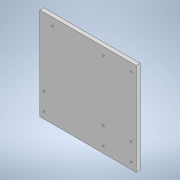
# Autodesk Inventor part: newMATXMount
Saved by Autodesk Inventor 2020 (Build 240168000, 168)
## iProperties
Created: 2026-07-11
Part Number: newMATXMount
Material: Generic
Document SubType Name: Modeling
Designer: Nessa
Density: 1 g/cm^3
Appearance: Default
Author: Nessa
Autodesk Inventor part; units mm, degrees
ref_plane "YZ Plane" through (0, 0, 0) normal (1, 0, 0) x (0, 1, 0)
ref_plane "XZ Plane" through (0, 0, 0) normal (0, 1, 0) x (-1, 0, 0)
ref_plane "XY Plane" through (0, 0, 0) normal (0, 0, 1) x (1, 0, 0)
sketch "Sketch1" plane through (0, 0, 0) normal (0, 0, 1) x (1, 0, 0)
  line L0 (-125, 120) -> (125, 120)
  line L1 (125, 120) -> (125, -120)
  line L2 (125, -120) -> (-125, -120)
  line L3 (-125, -120) -> (-125, 120)
  point P0 (0, 0)
  dimension "d0" = 250
  dimension "d1" = 240
  dimension "d2" = 125
  dimension "d3" = 120
  constraints: 8 end point, 2 parallel, 1 horizontal, 1 perpendicular
  measures "d0" distance of L1.end L2.end
  measures "d1" distance of L0.end L1.end
  measures "d2" distance from line of L3 point (0, 0)
  measures "d3" distance from line of L0 point (0, 0)
extrude "Extrusion1" add sketch "Sketch1" along normal mid plane 10
sketch "Sketch5" plane through (0, 0, 5) normal (0, 0, 1) x (1, 0, 0)
  line L0 (-115, 100) -> (-115, -103.2)
  line L1 (-92.14, 100) -> (-92.14, -103.2)
  line L2 (39.94, 100) -> (39.94, -103.2)
  line L3 (112.33, 100) -> (112.33, -103.2)
  line L4 (-92.14, 100) -> (112.33, 100)
  line L5 (-115, -57.48) -> (39.94, -57.48)
  line L6 (112.33, -57.48) -> (39.94, -57.48)
  line L7 (-115, -103.2) -> (39.94, -103.2)
  line L8 (112.33, -103.2) -> (39.94, -103.2)
  line L9 (-115, 100) -> (-92.14, 100)
  line L10 (-125, 120) -> (-125, -120) projected
  line L11 (125, 120) -> (-125, 120) projected
  point P0 (0, 0)
  dimension "d25" = 10
  dimension "d26" = 22.86
  dimension "d27" = 72.39
  dimension "d28" = 132.08
  dimension "d29" = 45.72
  dimension "d30" = 157.48
  dimension "d38" = 20
  constraints: 20 end point, 6 point on line, 4 perpendicular, 4 vertical, 2 collinear, 1 horizontal, 1 parallel
  measures "d25" distance between parallel lines of L10 L0
  measures "d26" distance between parallel lines of L1 L0
  measures "d27" distance between parallel lines of L3 L2
  measures "d28" distance between parallel lines of L2 L1
  measures "d29" distance between parallel lines of L8 L6
  measures "d30" distance between parallel lines of L4 L6
  measures "d38" distance between parallel lines of L11 L4
hole "Hole2" at (-92.14, 100, 5) at (39.94, 100, 5) at (112.33, 100, 5) at (112.33, -57.48, 5) at (39.94, -57.48, 5) at (39.94, -103.2, 5) at (112.33, -103.2, 5) at (-115, -57.48, 5) at (-115, -103.2, 5) direction (0, 0, -1) diameter 3.6 depth 5 tip angle 118
equation "\"d2\" = 0.5 * d0"
equation "\"d3\" = 0.5 * d1"
body "Solid1"
